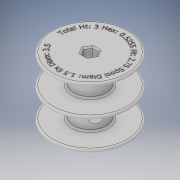
# Autodesk Inventor part: spoolV01
Saved by Autodesk Inventor 2019.3 (Build 233278000, 278)
## iProperties
Created: 2019-02-25
Part Number: spoolV01
Material: Generic
Document SubType Name: Modeling
Designer: steele
Density: 1 g/cm^3
Appearance: Default
d0: 2.750 in
d1: 0.150 in
d2: 0.750 in
d3: 1.750 in
d4: 0.075 in
d5: 0.075 in
d8: 0.523 in
d10: 0.00 deg
d17: 0.575 in
d18: 0.575 in
d19: 0.200 in
d20: 0.361 in
d21: 0.361 in
d23: 0.00 deg
d30: 2.625 in
d31: 0.050 in
d32: 0.00 deg
d33: 0.188 in
d36: 0.950 in
d37: 0.250 in
d38: 0.00 deg
d39: 0.063 in
holeForString: 0.200 in
stringDiameter: 0.120 in
clearanceForString: 0.080 in
hexShaftDiameter: 0.500 in
clearanceForHexShaft: 0.023 in
hexDiameter: 0.523 in
supportChannels: 0.150 in
spoolInteriorDiameter: 1.500 in
spoolInteriroRadius: 0.750 in
spoolExteriorDiameter: 3.500 in
spoolExteriorRadius: 1.750 in
spoolFiletRadius: 0.075 in
holeCenter: 0.575 in
hexHoleChamfer: 0.063 in
stringHoleCenterFromHexShaft: 0.361 in
textCircleDiameter: 2.625 in
textHeight: 0.240 in
textDepth: 0.050 in
stringHoleChamfer: 0.188 in
spoolTotalHeight: 3.000 in
spaceHeight: 0.250 in
spacerDiameter: 0.950 in
spoolHeightWithoutSpacer: 2.750 in
Author: steele
Autodesk Inventor part; units mm, degrees
(part 1 of 2)
ref_plane "YZ Plane" through (0, 0, 0) normal (1, 0, 0) x (0, 1, 0)
ref_plane "XZ Plane" through (0, 0, 0) normal (0, 1, 0) x (-1, 0, 0)
sketch "Sketch1" plane through (0, 0, 0) normal (1, 0, 0) x (0, 1, 0)
  line L0 (0, 0) -> (0, -42.545)
  line L1 (1.905, -44.45) -> (1.905, -44.45)
  line L2 (3.81, -42.545) -> (3.81, -20.955)
  line L3 (5.715, -19.05) -> (31.115, -19.05)
  line L4 (33.02, -20.955) -> (33.02, -42.545)
  line L5 (34.925, -44.45) -> (34.925, -44.45)
  line L6 (36.83, -42.545) -> (36.83, -20.955)
  line L7 (38.735, -19.05) -> (64.135, -19.05)
  line L8 (66.04, -20.955) -> (66.04, -42.545)
  line L9 (67.945, -44.45) -> (67.945, -44.45)
  line L10 (69.85, -42.545) -> (69.85, 0)
  line L11 (0, 0) -> (69.85, 0)
  arc A0 (67.945, -44.45) -> (69.85, -42.545) centre (67.945, -42.545) ccw
  arc A1 (66.04, -42.545) -> (67.945, -44.45) centre (67.945, -42.545) ccw
  arc A2 (34.925, -44.45) -> (36.83, -42.545) centre (34.925, -42.545) ccw
  arc A3 (33.02, -42.545) -> (34.925, -44.45) centre (34.925, -42.545) ccw
  arc A4 (1.905, -44.45) -> (3.81, -42.545) centre (1.905, -42.545) ccw
  arc A5 (0, -42.545) -> (1.905, -44.45) centre (1.905, -42.545) ccw
  arc A6 (66.04, -20.955) -> (64.135, -19.05) centre (64.135, -20.955) ccw
  arc A7 (38.735, -19.05) -> (36.83, -20.955) centre (38.735, -20.955) ccw
  arc A8 (33.02, -20.955) -> (31.115, -19.05) centre (31.115, -20.955) ccw
  arc A9 (5.715, -19.05) -> (3.81, -20.955) centre (5.715, -20.955) ccw
  point P0 (66.04, -44.45)
  point P1 (69.85, -44.45)
  dimension "d0" = 69.85
  dimension "d1" = 3.81
  dimension "d2" = 19.05
  dimension "d3" = 44.45
  dimension "d4" = 1.905
  dimension "d5" = 1.905
  constraints: 24 end point, 20 point on circle, 20 tangent, 10 centre point, 8 equal radius, 6 perpendicular, 6 point on line, 5 collinear, 1 horizontal, 1 parallel, 1 vertical
  measures "d0" distance between parallel lines of L10 L0
  measures "d1" distance of point (66.04, -44.45) point (69.85, -44.45)
  measures "d2" distance between parallel lines of L3 L11
  measures "d3" distance between parallel lines of L1 L11
  measures "d4" radius of A0
  measures "d5" radius of A6
revolve "Revolution1" add sketch "Sketch1" angle 360 about axis through (0, 0, 0) along (0, 1, 0)
sketch "Sketch6" plane through (0, 0, 0) normal (0, -1, 0) x (1, 0, 0)
  circle A0 centre (0, 0) radius 12.065
  dimension "d36" = 24.13
  constraints: 1 centre point, 1 coincident
  measures "d36" diameter of A0
extrude "Spacer" add sketch "Sketch6" along normal blind 6.35
sketch "Sketch2" plane through (0, 69.85, 0) normal (0, 1, 0) x (1, 0, 0)
  line L0 (7.6623, 0) -> (3.8312, -6.6357)
  line L1 (3.8312, -6.6357) -> (-3.8312, -6.6357)
  line L2 (-3.8312, -6.6357) -> (-7.6623, 0)
  line L3 (-7.6623, 0) -> (-3.8312, 6.6357)
  line L4 (-3.8312, 6.6357) -> (3.8312, 6.6358)
  line L5 (3.8312, 6.6358) -> (7.6623, 0)
  point P0 (0, 0)
  point P1 (0, 0)
  dimension "d8" = 13.2715
  constraints: 12 end point, 1 coincident, 1 horizontal, 13 other
  measures "d8" distance between parallel lines of L1 L4
extrude "HexHole" cut sketch "Sketch2" along normal through all both and the other way through all
sketch "Sketch4" plane through (0, 0, 0) normal (1, 0, 0) x (0, 1, 0)
  circle A0 centre (51.435, 9.1758) radius 2.54
  circle A1 centre (18.415, 9.1758) radius 2.54
  line L0 (3.81, 42.545) -> (3.81, -42.545) projected
  line L1 (66.04, 42.545) -> (66.04, -42.545) projected
  line L2 (69.85, 0) -> (0, 0) projected
  dimension "d17" = 14.605
  dimension "d18" = 14.605
  dimension "d19" = 5.08
  dimension "d20" = 9.1758
  dimension "d21" = 9.1758
  constraints: 2 centre point, 1 equal radius
  measures "d17" distance from line of A1.centre L0
  measures "d18" distance from line of A0.centre L1
  measures "d19" diameter of A0
  measures "d20" distance from line of A1.centre L2
  measures "d21" distance from line of A0.centre L2
extrude "StringHoles" cut sketch "Sketch4" along normal through all both and the other way through all
sketch "Sketch5" plane through (0, 69.85, 0) normal (0, 1, 0) x (1, 0, 0)
  circle A0 centre (0, 0) radius 33.3375
  line L0 (-33.296, 1.697) -> (-37.7666, 1.9708)
  line L1 (-37.7666, 1.9708) -> (-37.8708, 0.2697)
  line L2 (-37.8708, 0.2697) -> (-38.4707, 0.3065)
  line L3 (-38.4707, 0.3065) -> (-38.2211, 4.3826)
  line L4 (-38.2211, 4.3826) -> (-37.6212, 4.3458)
  line L5 (-37.6212, 4.3458) -> (-37.7253, 2.6447)
  line L6 (-37.7253, 2.6447) -> (-33.2548, 2.3709)
  line L7 (-33.2548, 2.3709) -> (-33.296, 1.697)
  spline S0 degree 2 poles (-34.3762, 7.9551) (-33.4283, 7.7835) (-32.5604, 6.685) (-32.6983, 5.9234) knots 0 0 0 1 2 2 2
  spline S1 degree 2 poles (-32.6983, 5.9234) (-32.8398, 5.1416) (-34.0673, 4.4393) (-34.9828, 4.6051) knots 0 0 0 1 2 2 2
  spline S2 degree 2 poles (-34.9828, 4.6051) (-35.9226, 4.7753) (-36.7964, 5.8874) (-36.66, 6.6408) knots 0 0 0 1 2 2 2
  spline S3 degree 2 poles (-36.66, 6.6408) (-36.5221, 7.4024) (-35.32, 8.126) (-34.3762, 7.9551) knots 0 0 0 1 2 2 2
  spline S4 degree 2 poles (-34.4943, 7.3029) (-35.2234, 7.435) (-36.0284, 7.0327) (-36.1172, 6.5425) knots 0 0 0 1 2 2 2
  spline S5 degree 2 poles (-36.1172, 6.5425) (-36.2059, 6.0524) (-35.5939, 5.3893) (-34.8647, 5.2573) knots 0 0 0 1 2 2 2
  spline S6 degree 2 poles (-34.8647, 5.2573) (-34.1558, 5.1289) (-33.3298, 5.5316) (-33.2411, 6.0217) knots 0 0 0 1 2 2 2
  spline S7 degree 2 poles (-33.2411, 6.0217) (-33.1531, 6.5078) (-33.7732, 7.1724) (-34.4943, 7.3029) knots 0 0 0 1 2 2 2
  spline S8 degree 2 poles (-31.9292, 9.337) (-32.0692, 8.8333) (-32.8019, 8.4259) (-33.4246, 8.5989) knots 0 0 0 1 2 2 2
  line L8 (-33.4246, 8.5989) -> (-35.4594, 9.1643)
  line L9 (-35.4594, 9.1643) -> (-35.5751, 8.7478)
  line L10 (-35.5751, 8.7478) -> (-36.0868, 8.89)
  line L11 (-36.0868, 8.89) -> (-35.9711, 9.3064)
  line L12 (-35.9711, 9.3064) -> (-37.0262, 9.5996)
  line L13 (-37.0262, 9.5996) -> (-36.8542, 10.2183)
  line L14 (-36.8542, 10.2183) -> (-35.7992, 9.9252)
  line L15 (-35.7992, 9.9252) -> (-35.4829, 11.0636)
  line L16 (-35.4829, 11.0636) -> (-34.9712, 10.9214)
  line L17 (-34.9712, 10.9214) -> (-35.2875, 9.783)
  line L18 (-35.2875, 9.783) -> (-33.5383, 9.297)
  spline S9 degree 2 poles (-33.5383, 9.297) (-33.2606, 9.2199) (-32.9497, 9.1549) (-32.8001, 9.1859) knots 0 0 0 1 2 2 2
  spline S10 degree 2 poles (-32.8001, 9.1859) (-32.6696, 9.2095) (-32.4852, 9.4274) (-32.4257, 9.6416) knots 0 0 0 1 2 2 2
  spline S11 degree 2 poles (-32.4257, 9.6416) (-32.3838, 9.7923) (-32.3968, 10.0993) (-32.4069, 10.1705) knots 0 0 0 1 2 2 2
  line L19 (-32.4069, 10.1705) -> (-32.397, 10.2062)
  line L20 (-32.397, 10.2062) -> (-31.8417, 10.0519)
  spline S12 degree 2 poles (-31.8417, 10.0519) (-31.8426, 9.8641) (-31.8862, 9.4917) (-31.9292, 9.337) knots 0 0 0 1 2 2 2
  spline S13 degree 2 poles (-31.2991, 12.625) (-31.2728, 12.5315) (-31.1733, 12.2123) (-31.1591, 12.0749) knots 0 0 0 1 2 2 2
  spline S14 degree 2 poles (-31.1591, 12.0749) (-31.134, 11.885) (-31.1574, 11.555) (-31.2592, 11.2854) knots 0 0 0 1 2 2 2
  spline S15 degree 2 poles (-31.2592, 11.2854) (-31.3421, 11.0659) (-31.6575, 10.7318) (-31.8644, 10.6383) knots 0 0 0 1 2 2 2
  spline S16 degree 2 poles (-31.8644, 10.6383) (-32.0645, 10.551) (-32.5613, 10.5406) (-32.8001, 10.6307) knots 0 0 0 1 2 2 2
  spline S17 degree 2 poles (-32.8001, 10.6307) (-33.1698, 10.7703) (-33.5758, 11.2801) (-33.598, 11.6757) knots 0 0 0 1 2 2 2
  spline S18 degree 2 poles (-33.598, 11.6757) (-33.6233, 12.0284) (-33.419, 12.8842) (-33.2671, 13.3681) knots 0 0 0 1 2 2 2
  line L21 (-33.2671, 13.3681) -> (-33.3826, 13.4117)
  spline S19 degree 2 poles (-33.3826, 13.4117) (-33.5906, 13.4902) (-33.8966, 13.4605) (-34.0134, 13.3726) knots 0 0 0 1 2 2 2
  spline S20 degree 2 poles (-34.0134, 13.3726) (-34.1302, 13.2847) (-34.3015, 12.971) (-34.3684, 12.7938) knots 0 0 0 1 2 2 2
  spline S21 degree 2 poles (-34.3684, 12.7938) (-34.4469, 12.5858) (-34.536, 11.977) (-34.5227, 11.6508) knots 0 0 0 1 2 2 2
  line L22 (-34.5227, 11.6508) -> (-34.5358, 11.6161)
  line L23 (-34.5358, 11.6161) -> (-35.1482, 11.8473)
  spline S22 degree 2 poles (-35.1482, 11.8473) (-35.1319, 12.0304) (-35.0133, 12.6941) (-34.8984, 12.9983) knots 0 0 0 1 2 2 2
  spline S23 degree 2 poles (-34.8984, 12.9983) (-34.7588, 13.3681) (-34.4528, 13.8289) (-34.227, 13.9725) knots 0 0 0 1 2 2 2
  spline S24 degree 2 poles (-34.227, 13.9725) (-34.0064, 14.1137) (-33.4677, 14.1303) (-33.1327, 14.0038) knots 0 0 0 1 2 2 2
  line L24 (-33.1327, 14.0038) -> (-30.6948, 13.0833)
  line L25 (-30.6948, 13.0833) -> (-30.9216, 12.4825)
  line L26 (-30.9216, 12.4825) -> (-31.2991, 12.625)
  line L27 (-31.7997, 12.814) -> (-32.7895, 13.1878)
  spline S25 degree 2 poles (-32.7895, 13.1878) (-32.8517, 12.9648) (-33.032, 12.2892) (-33.0474, 12.0618) knots 0 0 0 1 2 2 2
  spline S26 degree 2 poles (-33.0474, 12.0618) (-33.0644, 11.7954) (-32.8779, 11.3686) (-32.6083, 11.2668) knots 0 0 0 1 2 2 2
  spline S27 degree 2 poles (-32.6083, 11.2668) (-32.3002, 11.1505) (-31.8574, 11.3793) (-31.7323, 11.7105) knots 0 0 0 1 2 2 2
  spline S28 degree 2 poles (-31.7323, 11.7105) (-31.6262, 11.9917) (-31.6943, 12.5454) (-31.7997, 12.814) knots 0 0 0 1 2 2 2
  line L28 (-30.0264, 14.4882) -> (-30.2999, 13.9071)
  line L29 (-30.2999, 13.9071) -> (-35.1011, 16.167)
  line L30 (-35.1011, 16.167) -> (-34.8276, 16.748)
  line L31 (-34.8276, 16.748) -> (-30.0264, 14.4882)
  line L32 (-26.4744, 20.3444) -> (-26.8556, 19.7872)
  line L33 (-26.8556, 19.7872) -> (-28.9078, 21.1911)
  line L34 (-28.9078, 21.1911) -> (-30.228, 19.2611)
  line L35 (-30.228, 19.2611) -> (-28.1758, 17.8573)
  line L36 (-28.1758, 17.8573) -> (-28.5569, 17.3)
  line L37 (-28.5569, 17.3) -> (-32.7498, 20.1682)
  line L38 (-32.7498, 20.1682) -> (-32.3686, 20.7254)
  line L39 (-32.3686, 20.7254) -> (-30.7241, 19.6005)
  line L40 (-30.7241, 19.6005) -> (-29.4039, 21.5304)
  line L41 (-29.4039, 21.5304) -> (-31.0484, 22.6554)
  line L42 (-31.0484, 22.6554) -> (-30.6673, 23.2126)
  line L43 (-30.6673, 23.2126) -> (-26.4744, 20.3444)
  spline S29 degree 2 poles (-25.029, 21.9136) (-25.3681, 21.5156) (-26.2042, 21.4546) (-26.6962, 21.8738) knots 0 0 0 1 2 2 2
  line L44 (-26.6962, 21.8738) -> (-28.3037, 23.2433)
  line L45 (-28.3037, 23.2433) -> (-28.5841, 22.9143)
  line L46 (-28.5841, 22.9143) -> (-28.9883, 23.2587)
  line L47 (-28.9883, 23.2587) -> (-28.708, 23.5877)
  line L48 (-28.708, 23.5877) -> (-29.5415, 24.2979)
  line L49 (-29.5415, 24.2979) -> (-29.125, 24.7867)
  line L50 (-29.125, 24.7867) -> (-28.2915, 24.0766)
  line L51 (-28.2915, 24.0766) -> (-27.5253, 24.9759)
  line L52 (-27.5253, 24.9759) -> (-27.121, 24.6315)
  line L53 (-27.121, 24.6315) -> (-27.8872, 23.7322)
  line L54 (-27.8872, 23.7322) -> (-26.5053, 22.5548)
  spline S30 degree 2 poles (-26.5053, 22.5548) (-26.286, 22.3679) (-26.0313, 22.178) (-25.8825, 22.1432) knots 0 0 0 1 2 2 2
  spline S31 degree 2 poles (-25.8825, 22.1432) (-25.7543, 22.1097) (-25.4952, 22.2296) (-25.3511, 22.3989) knots 0 0 0 1 2 2 2
  spline S32 degree 2 poles (-25.3511, 22.3989) (-25.2496, 22.5179) (-25.1321, 22.8018) (-25.1113, 22.8707) knots 0 0 0 1 2 2 2
  line L55 (-25.1113, 22.8707) -> (-25.0873, 22.8989)
  line L56 (-25.0873, 22.8989) -> (-24.6486, 22.5251)
  spline S33 degree 2 poles (-24.6486, 22.5251) (-24.7285, 22.3552) (-24.9249, 22.0358) (-25.029, 21.9136) knots 0 0 0 1 2 2 2
  line L57 (-23.4674, 23.6819) -> (-24.0394, 23.1012)
  line L58 (-24.0394, 23.1012) -> (-24.7316, 23.7829)
  line L59 (-24.7316, 23.7829) -> (-24.1597, 24.3636)
  line L60 (-24.1597, 24.3636) -> (-23.4674, 23.6819)
  line L61 (-25.4913, 25.675) -> (-26.0633, 25.0943)
  line L62 (-26.0633, 25.0943) -> (-26.7555, 25.7759)
  line L63 (-26.7555, 25.7759) -> (-26.1836, 26.3567)
  line L64 (-26.1836, 26.3567) -> (-25.4913, 25.675)
  spline S34 degree 2 poles (-22.5898, 30.4771) (-22.7391, 30.3675) (-22.9808, 30.0776) (-23.0821, 29.9164) knots 0 0 0 1 2 2 2
  spline S35 degree 2 poles (-23.0821, 29.9164) (-23.1733, 29.7625) (-23.2814, 29.4993) (-23.3187, 29.3901) knots 0 0 0 1 2 2 2
  line L65 (-23.3187, 29.3901) -> (-23.3519, 29.3658)
  line L66 (-23.3519, 29.3658) -> (-23.7783, 29.9464)
  spline S36 degree 2 poles (-23.7783, 29.9464) (-23.6698, 30.1742) (-23.1706, 30.781) (-22.8952, 30.9833) knots 0 0 0 1 2 2 2
  spline S37 degree 2 poles (-22.8952, 30.9833) (-22.6165, 31.188) (-22.1189, 31.3798) (-21.862, 31.3846) knots 0 0 0 1 2 2 2
  spline S38 degree 2 poles (-21.862, 31.3846) (-21.5877, 31.3868) (-21.1266, 31.1484) (-20.9414, 30.8962) knots 0 0 0 1 2 2 2
  spline S39 degree 2 poles (-20.9414, 30.8962) (-20.6928, 30.5578) (-20.7621, 29.7203) (-21.0252, 29.4249) knots 0 0 0 1 2 2 2
  line L67 (-21.0252, 29.4249) -> (-20.996, 29.385)
  spline S40 degree 2 poles (-20.996, 29.385) (-20.8471, 29.4535) (-20.4641, 29.551) (-20.2503, 29.5241) knots 0 0 0 1 2 2 2
  spline S41 degree 2 poles (-20.2503, 29.5241) (-20.0389, 29.5006) (-19.6067, 29.246) (-19.4093, 28.9773) knots 0 0 0 1 2 2 2
  spline S42 degree 2 poles (-19.4093, 28.9773) (-19.207, 28.7019) (-19.0525, 28.0951) (-19.0935, 27.7893) knots 0 0 0 1 2 2 2
  spline S43 degree 2 poles (-19.0935, 27.7893) (-19.1361, 27.4719) (-19.5024, 26.9066) (-19.8243, 26.6702) knots 0 0 0 1 2 2 2
  spline S44 degree 2 poles (-19.8243, 26.6702) (-20.1328, 26.4435) (-20.8463, 26.1493) (-21.1276, 26.1011) knots 0 0 0 1 2 2 2
  line L68 (-21.1276, 26.1011) -> (-21.5541, 26.6817)
  line L69 (-21.5541, 26.6817) -> (-21.5143, 26.7109)
  spline S45 degree 2 poles (-21.5143, 26.7109) (-21.2491, 26.7116) (-20.4946, 26.9082) (-20.2059, 27.1203) knots 0 0 0 1 2 2 2
  spline S46 degree 2 poles (-20.2059, 27.1203) (-20.0367, 27.2445) (-19.7763, 27.5993) (-19.7536, 27.8049) knots 0 0 0 1 2 2 2
  spline S47 degree 2 poles (-19.7536, 27.8049) (-19.7343, 28.0081) (-19.8327, 28.3854) (-19.9959, 28.6077) knots 0 0 0 1 2 2 2
  spline S48 degree 2 poles (-19.9959, 28.6077) (-20.1592, 28.83) (-20.5006, 29.0236) (-20.6777, 29.0212) knots 0 0 0 1 2 2 2
  spline S49 degree 2 poles (-20.6777, 29.0212) (-20.8547, 29.0189) (-21.2162, 28.8504) (-21.402, 28.7139) knots 0 0 0 1 2 2 2
  line L70 (-21.402, 28.7139) -> (-21.6343, 28.5433)
  line L71 (-21.6343, 28.5433) -> (-21.9681, 28.9979)
  line L72 (-21.9681, 28.9979) -> (-21.7857, 29.1319)
  spline S50 degree 2 poles (-21.7857, 29.1319) (-21.4174, 29.4024) (-21.2112, 30.0953) (-21.4573, 30.4304) knots 0 0 0 1 2 2 2
  spline S51 degree 2 poles (-21.4573, 30.4304) (-21.5719, 30.5863) (-21.8546, 30.7209) (-21.9995, 30.7166) knots 0 0 0 1 2 2 2
  spline S52 degree 2 poles (-21.9995, 30.7166) (-22.1536, 30.7107) (-22.4472, 30.5819) (-22.5898, 30.4771) knots 0 0 0 1 2 2 2
  line L73 (-12.5415, 30.9435) -> (-13.1522, 30.6558)
  line L74 (-13.1522, 30.6558) -> (-14.2121, 32.905)
  line L75 (-14.2121, 32.905) -> (-16.3273, 31.9084)
  line L76 (-16.3273, 31.9084) -> (-15.2674, 29.6591)
  line L77 (-15.2674, 29.6591) -> (-15.8782, 29.3713)
  line L78 (-15.8782, 29.3713) -> (-18.0435, 33.9667)
  line L79 (-18.0435, 33.9667) -> (-17.4327, 34.2545)
  line L80 (-17.4327, 34.2545) -> (-16.5835, 32.4521)
  line L81 (-16.5835, 32.4521) -> (-14.4682, 33.4488)
  line L82 (-14.4682, 33.4488) -> (-15.3175, 35.2512)
  line L83 (-15.3175, 35.2512) -> (-14.7068, 35.5389)
  line L84 (-14.7068, 35.5389) -> (-12.5415, 30.9435)
  spline S53 degree 2 poles (-10.0214, 31.7062) (-10.8904, 31.4234) (-12.1628, 32.0873) (-12.4558, 32.9877) knots 0 0 0 1 2 2 2
  spline S54 degree 2 poles (-12.4558, 32.9877) (-12.7437, 33.8724) (-12.1573, 35.2234) (-11.4096, 35.4667) knots 0 0 0 1 2 2 2
  spline S55 degree 2 poles (-11.4096, 35.4667) (-11.073, 35.5763) (-10.4886, 35.55) (-10.2293, 35.4049) knots 0 0 0 1 2 2 2
  spline S56 degree 2 poles (-10.2293, 35.4049) (-9.9661, 35.2612) (-9.5637, 34.7297) (-9.4223, 34.2952) knots 0 0 0 1 2 2 2
  line L85 (-9.4223, 34.2952) -> (-9.314, 33.9625)
  line L86 (-9.314, 33.9625) -> (-11.8233, 33.1459)
  spline S57 degree 2 poles (-11.8233, 33.1459) (-11.6182, 32.5156) (-10.7662, 32.0526) (-10.2024, 32.2361) knots 0 0 0 1 2 2 2
  spline S58 degree 2 poles (-10.2024, 32.2361) (-10.0028, 32.301) (-9.6446, 32.5172) (-9.5109, 32.6386) knots 0 0 0 1 2 2 2
  spline S59 degree 2 poles (-9.5109, 32.6386) (-9.372, 32.7704) (-9.1895, 32.9813) (-9.1355, 33.0681) knots 0 0 0 1 2 2 2
  line L87 (-9.1355, 33.0681) -> (-9.1003, 33.0796)
  line L88 (-9.1003, 33.0796) -> (-8.8837, 32.4141)
  spline S60 degree 2 poles (-8.8837, 32.4141) (-8.9754, 32.3367) (-9.2556, 32.1069) (-9.3694, 32.0309) knots 0 0 0 1 2 2 2
  spline S61 degree 2 poles (-9.3694, 32.0309) (-9.529, 31.9227) (-9.8021, 31.7776) (-10.0214, 31.7062) knots 0 0 0 1 2 2 2
  spline S62 degree 2 poles (-10.0606, 34.2347) (-10.1487, 34.4788) (-10.3677, 34.8058) (-10.505, 34.8953) knots 0 0 0 1 2 2 2
  spline S63 degree 2 poles (-10.505, 34.8953) (-10.6553, 34.9979) (-11.0352, 35.0345) (-11.2818, 34.9542) knots 0 0 0 1 2 2 2
  spline S64 degree 2 poles (-11.2818, 34.9542) (-11.5245, 34.8752) (-11.818, 34.6195) (-11.913, 34.4328) knots 0 0 0 1 2 2 2
  spline S65 degree 2 poles (-11.913, 34.4328) (-12.0029, 34.2433) (-12.0304, 33.8491) (-11.9749, 33.6117) knots 0 0 0 1 2 2 2
  line L89 (-11.9749, 33.6117) -> (-10.0606, 34.2347)
  line L90 (-5.2154, 32.9707) -> (-5.9848, 32.8085)
  line L91 (-5.9848, 32.8085) -> (-7.1866, 34.0193)
  line L92 (-7.1866, 34.0193) -> (-7.8217, 32.4214)
  line L93 (-7.8217, 32.4214) -> (-8.5347, 32.2711)
  line L94 (-8.5347, 32.2711) -> (-7.6313, 34.3926)
  line L95 (-7.6313, 34.3926) -> (-9.3087, 36.0038)
  line L96 (-9.3087, 36.0038) -> (-8.5393, 36.1659)
  line L97 (-8.5393, 36.1659) -> (-7.3441, 34.9664)
  line L98 (-7.3441, 34.9664) -> (-6.7146, 36.5505)
  line L99 (-6.7146, 36.5505) -> (-6.0016, 36.7008)
  line L100 (-6.0016, 36.7008) -> (-6.8986, 34.5891)
  line L101 (-6.8986, 34.5891) -> (-5.2154, 32.9707)
  line L102 (-3.5488, 33.1506) -> (-4.3582, 33.0539)
  line L103 (-4.3582, 33.0539) -> (-4.4734, 34.0186)
  line L104 (-4.4734, 34.0186) -> (-3.664, 34.1153)
  line L105 (-3.664, 34.1153) -> (-3.5488, 33.1506)
  line L106 (-3.8857, 35.9711) -> (-4.695, 35.8744)
  line L107 (-4.695, 35.8744) -> (-4.8103, 36.8391)
  line L108 (-4.8103, 36.8391) -> (-4.0009, 36.9357)
  line L109 (-4.0009, 36.9357) -> (-3.8857, 35.9711)
  spline S66 degree 2 poles (3.0843, 35.7816) (3.0287, 34.416) (2.1828, 33.1691) (1.356, 33.2028) knots 0 0 0 1 2 2 2
  spline S67 degree 2 poles (1.356, 33.2028) (0.5169, 33.237) (-0.2156, 34.5729) (-0.1612, 35.9097) knots 0 0 0 1 2 2 2
  spline S68 degree 2 poles (-0.1612, 35.9097) (-0.1053, 37.2835) (0.7404, 38.5222) (1.5712, 38.4884) knots 0 0 0 1 2 2 2
  spline S69 degree 2 poles (1.5712, 38.4884) (2.4062, 38.4544) (3.1383, 37.1061) (3.0843, 35.7816) knots 0 0 0 1 2 2 2
  spline S70 degree 2 poles (2.1494, 34.2706) (2.2583, 34.5174) (2.372, 35.2874) (2.3933, 35.8098) knots 0 0 0 1 2 2 2
  spline S71 degree 2 poles (2.3933, 35.8098) (2.4146, 36.3322) (2.3636, 37.1047) (2.2714, 37.368) knots 0 0 0 1 2 2 2
  spline S72 degree 2 poles (2.2714, 37.368) (2.1791, 37.6313) (1.8321, 37.9133) (1.5483, 37.9248) knots 0 0 0 1 2 2 2
  spline S73 degree 2 poles (1.5483, 37.9248) (1.2645, 37.9364) (0.8875, 37.6839) (0.7697, 37.4209) knots 0 0 0 1 2 2 2
  spline S74 degree 2 poles (0.7697, 37.4209) (0.6563, 37.166) (0.5501, 36.3792) (0.5298, 35.8815) knots 0 0 0 1 2 2 2
  spline S75 degree 2 poles (0.5298, 35.8815) (0.5081, 35.3468) (0.5447, 34.6284) (0.6403, 34.3444) knots 0 0 0 1 2 2 2
  spline S76 degree 2 poles (0.6403, 34.3444) (0.7283, 34.0771) (1.0828, 33.7784) (1.379, 33.7663) knots 0 0 0 1 2 2 2
  spline S77 degree 2 poles (1.379, 33.7663) (1.6587, 33.7549) (2.0356, 34.0074) (2.1494, 34.2706) knots 0 0 0 1 2 2 2
  line L110 (4.7062, 33.0061) -> (3.8979, 33.1114)
  line L111 (3.8979, 33.1114) -> (4.0234, 34.0748)
  line L112 (4.0234, 34.0748) -> (4.8317, 33.9695)
  line L113 (4.8317, 33.9695) -> (4.7062, 33.0061)
  spline S78 degree 2 poles (9.0788, 33.7868) (8.9994, 33.4291) (8.6348, 32.8691) (8.3759, 32.6904) knots 0 0 0 1 2 2 2
  spline S79 degree 2 poles (8.3759, 32.6904) (8.1169, 32.5117) (7.436, 32.3887) (7.0502, 32.4743) knots 0 0 0 1 2 2 2
  spline S80 degree 2 poles (7.0502, 32.4743) (6.6966, 32.5528) (6.0401, 32.8629) (5.8145, 33.0437) knots 0 0 0 1 2 2 2
  line L114 (5.8145, 33.0437) -> (5.9706, 33.747)
  line L115 (5.9706, 33.747) -> (6.0188, 33.7363)
  spline S81 degree 2 poles (6.0188, 33.7363) (6.0827, 33.6631) (6.3359, 33.4551) (6.4945, 33.3525) knots 0 0 0 1 2 2 2
  spline S82 degree 2 poles (6.4945, 33.3525) (6.6763, 33.2404) (6.9848, 33.0918) (7.1898, 33.0464) knots 0 0 0 1 2 2 2
  spline S83 degree 2 poles (7.1898, 33.0464) (7.3908, 33.0018) (7.8006, 33.0626) (7.9721, 33.189) knots 0 0 0 1 2 2 2
  spline S84 degree 2 poles (7.9721, 33.189) (8.1296, 33.3101) (8.3457, 33.6754) (8.4045, 33.9406) knots 0 0 0 1 2 2 2
  spline S85 degree 2 poles (8.4045, 33.9406) (8.4634, 34.2059) (8.3936, 34.5756) (8.2819, 34.7184) knots 0 0 0 1 2 2 2
  spline S86 degree 2 poles (8.2819, 34.7184) (8.1689, 34.8742) (7.7741, 35.0715) (7.5209, 35.1277) knots 0 0 0 1 2 2 2
  spline S87 degree 2 poles (7.5209, 35.1277) (7.2477, 35.1883) (6.6864, 35.2243) (6.5136, 35.2247) knots 0 0 0 1 2 2 2
  line L116 (6.5136, 35.2247) -> (7.0808, 37.7808)
  line L117 (7.0808, 37.7808) -> (9.8016, 37.177)
  line L118 (9.8016, 37.177) -> (9.6723, 36.5942)
  line L119 (9.6723, 36.5942) -> (7.5905, 37.0562)
  line L120 (7.5905, 37.0562) -> (7.2971, 35.734)
  spline S88 degree 2 poles (7.2971, 35.734) (7.4212, 35.7233) (7.657, 35.6836) (7.7534, 35.6622) knots 0 0 0 1 2 2 2
  spline S89 degree 2 poles (7.7534, 35.6622) (8.1352, 35.5775) (8.634, 35.3361) (8.8342, 35.0977) knots 0 0 0 1 2 2 2
  spline S90 degree 2 poles (8.8342, 35.0977) (9.0383, 34.8584) (9.1787, 34.2369) (9.0788, 33.7868) knots 0 0 0 1 2 2 2
  line L121 (12.3942, 30.9891) -> (9.4331, 32.0119)
  line L122 (9.4331, 32.0119) -> (9.6683, 32.6929)
  spline S91 degree 2 poles (9.6683, 32.6929) (10.0908, 32.8823) (10.8511, 33.2425) (11.227, 33.448) knots 0 0 0 1 2 2 2
  spline S92 degree 2 poles (11.227, 33.448) (11.984, 33.8616) (12.6348, 34.4469) (12.7678, 34.8321) knots 0 0 0 1 2 2 2
  spline S93 degree 2 poles (12.7678, 34.8321) (12.8377, 35.0345) (12.8181, 35.381) (12.7388, 35.5172) knots 0 0 0 1 2 2 2
  spline S94 degree 2 poles (12.7388, 35.5172) (12.6596, 35.6535) (12.3974, 35.8529) (12.2185, 35.9147) knots 0 0 0 1 2 2 2
  spline S95 degree 2 poles (12.2185, 35.9147) (12.0473, 35.9739) (11.6675, 36.0092) (11.4851, 35.9982) knots 0 0 0 1 2 2 2
  spline S96 degree 2 poles (11.4851, 35.9982) (11.3301, 35.9908) (11.0234, 35.9225) (10.9268, 35.8949) knots 0 0 0 1 2 2 2
  line L123 (10.9268, 35.8949) -> (10.8917, 35.907)
  line L124 (10.8917, 35.907) -> (11.1283, 36.5918)
  spline S97 degree 2 poles (11.1283, 36.5918) (11.3604, 36.6206) (12.1383, 36.5653) (12.4574, 36.455) knots 0 0 0 1 2 2 2
  spline S98 degree 2 poles (12.4574, 36.455) (13.1305, 36.2225) (13.6433, 35.2484) (13.4336, 34.6413) knots 0 0 0 1 2 2 2
  spline S99 degree 2 poles (13.4336, 34.6413) (13.3355, 34.3573) (13.0392, 33.9283) (12.8526, 33.7663) knots 0 0 0 1 2 2 2
  spline S100 degree 2 poles (12.8526, 33.7663) (12.6633, 33.5965) (12.1823, 33.3009) (11.927, 33.167) knots 0 0 0 1 2 2 2
  spline S101 degree 2 poles (11.927, 33.167) (11.5092, 32.9411) (10.5214, 32.4896) (10.2284, 32.36) knots 0 0 0 1 2 2 2
  line L125 (10.2284, 32.36) -> (12.5864, 31.5455)
  line L126 (12.5864, 31.5455) -> (12.3942, 30.9891)
  spline S102 degree 2 poles (16.4944, 30.853) (16.3361, 30.5226) (15.8541, 30.0596) (15.5615, 29.9442) knots 0 0 0 1 2 2 2
  spline S103 degree 2 poles (15.5615, 29.9442) (15.2688, 29.8288) (14.5777, 29.8632) (14.2213, 30.034) knots 0 0 0 1 2 2 2
  spline S104 degree 2 poles (14.2213, 30.034) (13.8946, 30.1905) (13.3254, 30.6413) (13.1467, 30.8684) knots 0 0 0 1 2 2 2
  line L127 (13.1467, 30.8684) -> (13.458, 31.5181)
  line L128 (13.458, 31.5181) -> (13.5025, 31.4968)
  spline S105 degree 2 poles (13.5025, 31.4968) (13.5482, 31.411) (13.7477, 31.1511) (13.8789, 31.0152) knots 0 0 0 1 2 2 2
  spline S106 degree 2 poles (13.8789, 31.0152) (14.0306, 30.8649) (14.2975, 30.6503) (14.4868, 30.5596) knots 0 0 0 1 2 2 2
  spline S107 degree 2 poles (14.4868, 30.5596) (14.6725, 30.4706) (15.0855, 30.4371) (15.2811, 30.5214) knots 0 0 0 1 2 2 2
  spline S108 degree 2 poles (15.2811, 30.5214) (15.462, 30.6036) (15.7551, 30.9105) (15.8725, 31.1555) knots 0 0 0 1 2 2 2
  spline S109 degree 2 poles (15.8725, 31.1555) (15.9899, 31.4006) (16.0057, 31.7764) (15.9293, 31.9409) knots 0 0 0 1 2 2 2
  spline S110 degree 2 poles (15.9293, 31.9409) (15.8545, 32.1182) (15.5146, 32.3997) (15.2807, 32.5118) knots 0 0 0 1 2 2 2
  spline S111 degree 2 poles (15.2807, 32.5118) (15.0283, 32.6328) (14.4897, 32.7949) (14.3215, 32.8345) knots 0 0 0 1 2 2 2
  line L129 (14.3215, 32.8345) -> (15.4528, 35.1956)
  line L130 (15.4528, 35.1956) -> (17.9662, 33.9914)
  line L131 (17.9662, 33.9914) -> (17.7083, 33.4531)
  line L132 (17.7083, 33.4531) -> (15.7852, 34.3745)
  line L133 (15.7852, 34.3745) -> (15.1999, 33.1531)
  spline S112 degree 2 poles (15.1999, 33.1531) (15.3184, 33.1146) (15.5391, 33.0225) (15.6282, 32.9798) knots 0 0 0 1 2 2 2
  spline S113 degree 2 poles (15.6282, 32.9798) (15.9809, 32.8108) (16.4121, 32.4627) (16.553, 32.1852) knots 0 0 0 1 2 2 2
  spline S114 degree 2 poles (16.553, 32.1852) (16.6977, 31.9059) (16.6937, 31.2688) (16.4944, 30.853) knots 0 0 0 1 2 2 2
  spline S115 degree 2 poles (19.9034, 28.772) (19.7085, 28.4618) (19.1769, 28.0568) (18.873, 27.9755) knots 0 0 0 1 2 2 2
  spline S116 degree 2 poles (18.873, 27.9755) (18.569, 27.8942) (17.8864, 28.0071) (17.5518, 28.2174) knots 0 0 0 1 2 2 2
  spline S117 degree 2 poles (17.5518, 28.2174) (17.245, 28.4102) (16.7309, 28.9228) (16.5792, 29.1689) knots 0 0 0 1 2 2 2
  line L134 (16.5792, 29.1689) -> (16.9626, 29.7789)
  line L135 (16.9626, 29.7789) -> (17.0044, 29.7526)
  spline S118 degree 2 poles (17.0044, 29.7526) (17.0399, 29.6622) (17.2086, 29.3812) (17.3234, 29.2312) knots 0 0 0 1 2 2 2
  spline S119 degree 2 poles (17.3234, 29.2312) (17.457, 29.0646) (17.6977, 28.821) (17.8755, 28.7093) knots 0 0 0 1 2 2 2
  spline S120 degree 2 poles (17.8755, 28.7093) (18.0497, 28.5998) (18.4562, 28.5194) (18.6602, 28.5808) knots 0 0 0 1 2 2 2
  spline S121 degree 2 poles (18.6602, 28.5808) (18.8493, 28.6419) (19.1755, 28.9134) (19.32, 29.1434) knots 0 0 0 1 2 2 2
  spline S122 degree 2 poles (19.32, 29.1434) (19.4646, 29.3735) (19.5231, 29.7451) (19.4659, 29.9172) knots 0 0 0 1 2 2 2
  spline S123 degree 2 poles (19.4659, 29.9172) (19.4118, 30.1019) (19.1063, 30.4203) (18.8867, 30.5583) knots 0 0 0 1 2 2 2
  spline S124 degree 2 poles (18.8867, 30.5583) (18.6496, 30.7073) (18.1331, 30.9298) (17.9705, 30.9882) knots 0 0 0 1 2 2 2
  line L136 (17.9705, 30.9882) -> (19.3635, 33.2051)
  line L137 (19.3635, 33.2051) -> (21.7233, 31.7222)
  line L138 (21.7233, 31.7222) -> (21.4057, 31.2168)
  line L139 (21.4057, 31.2168) -> (19.6001, 32.3514)
  line L140 (19.6001, 32.3514) -> (18.8795, 31.2046)
  spline S125 degree 2 poles (18.8795, 31.2046) (18.9928, 31.1528) (19.2016, 31.0363) (19.2852, 30.9837) knots 0 0 0 1 2 2 2
  spline S126 degree 2 poles (19.2852, 30.9837) (19.6164, 30.7756) (20.0051, 30.3806) (20.1135, 30.0889) knots 0 0 0 1 2 2 2
  spline S127 degree 2 poles (20.1135, 30.0889) (20.2253, 29.7949) (20.1487, 29.1624) (19.9034, 28.772) knots 0 0 0 1 2 2 2
  line L141 (24.1708, 23.034) -> (23.6787, 23.4962)
  line L142 (23.6787, 23.4962) -> (25.3813, 25.3084)
  line L143 (25.3813, 25.3084) -> (23.6771, 26.9095)
  line L144 (23.6771, 26.9095) -> (21.9746, 25.0973)
  line L145 (21.9746, 25.0973) -> (21.4825, 25.5596)
  line L146 (21.4825, 25.5596) -> (24.9609, 29.2619)
  line L147 (24.9609, 29.2619) -> (25.4529, 28.7996)
  line L148 (25.4529, 28.7996) -> (24.0886, 27.3475)
  line L149 (24.0886, 27.3475) -> (25.7928, 25.7465)
  line L150 (25.7928, 25.7465) -> (27.1571, 27.1986)
  line L151 (27.1571, 27.1986) -> (27.6491, 26.7363)
  line L152 (27.6491, 26.7363) -> (24.1708, 23.034)
  spline S128 degree 2 poles (25.4992, 21.3646) (25.158, 21.7608) (25.2263, 22.5964) (25.716, 23.0181) knots 0 0 0 1 2 2 2
  line L153 (25.716, 23.0181) -> (27.3164, 24.3961)
  line L154 (27.3164, 24.3961) -> (27.0343, 24.7237)
  line L155 (27.0343, 24.7237) -> (27.4367, 25.0702)
  line L156 (27.4367, 25.0702) -> (27.7188, 24.7426)
  line L157 (27.7188, 24.7426) -> (28.5486, 25.4572)
  line L158 (28.5486, 25.4572) -> (28.9676, 24.9705)
  line L159 (28.9676, 24.9705) -> (28.1378, 24.256)
  line L160 (28.1378, 24.256) -> (28.9088, 23.3607)
  line L161 (28.9088, 23.3607) -> (28.5063, 23.0142)
  line L162 (28.5063, 23.0142) -> (27.7354, 23.9095)
  line L163 (27.7354, 23.9095) -> (26.3597, 22.7249)
  spline S129 degree 2 poles (26.3597, 22.7249) (26.1413, 22.5368) (25.9145, 22.3144) (25.8572, 22.1727) knots 0 0 0 1 2 2 2
  spline S130 degree 2 poles (25.8572, 22.1727) (25.8044, 22.0512) (25.8831, 21.7767) (26.0282, 21.6083) knots 0 0 0 1 2 2 2
  spline S131 degree 2 poles (26.0282, 21.6083) (26.1303, 21.4897) (26.3927, 21.33) (26.4576, 21.2989) knots 0 0 0 1 2 2 2
  line L164 (26.4576, 21.2989) -> (26.4817, 21.2708)
  line L165 (26.4817, 21.2708) -> (26.045, 20.8948)
  spline S132 degree 2 poles (26.045, 20.8948) (25.8894, 20.9998) (25.6039, 21.243) (25.4992, 21.3646) knots 0 0 0 1 2 2 2
  line L166 (27.0066, 19.5499) -> (26.5206, 20.2042)
  line L167 (26.5206, 20.2042) -> (27.3006, 20.7835)
  line L168 (27.3006, 20.7835) -> (27.7866, 20.1291)
  line L169 (27.7866, 20.1291) -> (27.0066, 19.5499)
  line L170 (29.287, 21.2435) -> (28.801, 21.8979)
  line L171 (28.801, 21.8979) -> (29.581, 22.4771)
  line L172 (29.581, 22.4771) -> (30.067, 21.8228)
  line L173 (30.067, 21.8228) -> (29.287, 21.2435)
  line L174 (30.3184, 13.9548) -> (28.8738, 16.7347)
  line L175 (28.8738, 16.7347) -> (29.5131, 17.0669)
  spline S133 degree 2 poles (29.5131, 17.0669) (29.95, 16.9135) (30.7495, 16.6516) (31.1637, 16.5421) knots 0 0 0 1 2 2 2
  spline S134 degree 2 poles (31.1637, 16.5421) (31.9975, 16.3212) (32.8725, 16.2981) (33.2341, 16.486) knots 0 0 0 1 2 2 2
  spline S135 degree 2 poles (33.2341, 16.486) (33.4241, 16.5847) (33.6483, 16.8496) (33.6845, 17.003) knots 0 0 0 1 2 2 2
  spline S136 degree 2 poles (33.6845, 17.003) (33.7208, 17.1564) (33.6679, 17.4815) (33.5806, 17.6495) knots 0 0 0 1 2 2 2
  spline S137 degree 2 poles (33.5806, 17.6495) (33.497, 17.8103) (33.2458, 18.0973) (33.1059, 18.2148) knots 0 0 0 1 2 2 2
  spline S138 degree 2 poles (33.1059, 18.2148) (32.9883, 18.316) (32.7188, 18.4776) (32.6297, 18.524) knots 0 0 0 1 2 2 2
  line L176 (32.6297, 18.524) -> (32.6126, 18.5569)
  line L177 (32.6126, 18.5569) -> (33.2555, 18.891)
  spline S139 degree 2 poles (33.2555, 18.891) (33.4437, 18.7522) (33.97, 18.1767) (34.1257, 17.8771) knots 0 0 0 1 2 2 2
  spline S140 degree 2 poles (34.1257, 17.8771) (34.4541, 17.2452) (34.1558, 16.1855) (33.5859, 15.8894) knots 0 0 0 1 2 2 2
  spline S141 degree 2 poles (33.5859, 15.8894) (33.3192, 15.7508) (32.809, 15.6434) (32.5622, 15.6543) knots 0 0 0 1 2 2 2
  spline S142 degree 2 poles (32.5622, 15.6543) (32.3079, 15.6614) (31.7556, 15.778) (31.4782, 15.8565) knots 0 0 0 1 2 2 2
  spline S143 degree 2 poles (31.4782, 15.8565) (31.0196, 15.9801) (29.9922, 16.3323) (29.6904, 16.4399) knots 0 0 0 1 2 2 2
  line L178 (29.6904, 16.4399) -> (30.8407, 14.2262)
  line L179 (30.8407, 14.2262) -> (30.3184, 13.9548)
  line L180 (30.9826, 12.3139) -> (30.6724, 13.0677)
  line L181 (30.6724, 13.0677) -> (31.5708, 13.4374)
  line L182 (31.5708, 13.4374) -> (31.881, 12.6837)
  line L183 (31.881, 12.6837) -> (30.9826, 12.3139)
  line L184 (36.4481, 9.6043) -> (31.6716, 10.4207)
  line L185 (31.6716, 10.4207) -> (31.4564, 11.1126)
  line L186 (31.4564, 11.1126) -> (36.4268, 10.2271)
  line L187 (36.4268, 10.2271) -> (35.6479, 12.7311)
  line L188 (35.6479, 12.7311) -> (36.2179, 12.9084)
  line L189 (36.2179, 12.9084) -> (37.1753, 9.8305)
  line L190 (37.1753, 9.8305) -> (36.4481, 9.6043)
  spline S144 degree 2 poles (34.6272, 4.993) (34.2672, 4.9247) (33.6087, 5.0387) (33.3424, 5.2061) knots 0 0 0 1 2 2 2
  spline S145 degree 2 poles (33.3424, 5.2061) (33.076, 5.3735) (32.6942, 5.9506) (32.6206, 6.3389) knots 0 0 0 1 2 2 2
  spline S146 degree 2 poles (32.6206, 6.3389) (32.5532, 6.6948) (32.579, 7.4204) (32.6561, 7.699) knots 0 0 0 1 2 2 2
  line L191 (32.6561, 7.699) -> (33.3639, 7.8331)
  line L192 (33.3639, 7.8331) -> (33.3731, 7.7846)
  spline S147 degree 2 poles (33.3731, 7.7846) (33.3311, 7.697) (33.2399, 7.3823) (33.2081, 7.1961) knots 0 0 0 1 2 2 2
  spline S148 degree 2 poles (33.2081, 7.1961) (33.177, 6.9848) (33.1622, 6.6427) (33.2013, 6.4364) knots 0 0 0 1 2 2 2
  spline S149 degree 2 poles (33.2013, 6.4364) (33.2397, 6.2341) (33.4573, 5.8815) (33.6412, 5.7739) knots 0 0 0 1 2 2 2
  spline S150 degree 2 poles (33.6412, 5.7739) (33.8146, 5.6769) (34.2355, 5.6226) (34.5024, 5.6732) knots 0 0 0 1 2 2 2
  spline S151 degree 2 poles (34.5024, 5.6732) (34.7694, 5.7238) (35.0815, 5.9339) (35.1687, 6.0928) knots 0 0 0 1 2 2 2
  spline S152 degree 2 poles (35.1687, 6.0928) (35.2673, 6.2582) (35.2927, 6.6988) (35.2444, 6.9536) knots 0 0 0 1 2 2 2
  spline S153 degree 2 poles (35.2444, 6.9536) (35.1922, 7.2286) (35.0038, 7.7585) (34.936, 7.9175) knots 0 0 0 1 2 2 2
  line L193 (34.936, 7.9175) -> (37.5084, 8.4051)
  line L194 (37.5084, 8.4051) -> (38.0274, 5.6669)
  line L195 (38.0274, 5.6669) -> (37.441, 5.5557)
  line L196 (37.441, 5.5557) -> (37.0438, 7.6508)
  line L197 (37.0438, 7.6508) -> (35.7131, 7.3986)
  spline S154 degree 2 poles (35.7131, 7.3986) (35.7523, 7.2803) (35.8089, 7.048) (35.8273, 6.9509) knots 0 0 0 1 2 2 2
  spline S155 degree 2 poles (35.8273, 6.9509) (35.9001, 6.5667) (35.8752, 6.0131) (35.7351, 5.7351) knots 0 0 0 1 2 2 2
  spline S156 degree 2 poles (35.7351, 5.7351) (35.5958, 5.4531) (35.0802, 5.0788) (34.6272, 4.993) knots 0 0 0 1 2 2 2
  spline S157 degree 2 poles (33.2461, 0.2315) (33.2425, 0.7831) (33.468, 1.5585) (33.6304, 1.9013) knots 0 0 0 1 2 2 2
  line L198 (33.6304, 1.9013) -> (34.4785, 1.9068)
  line L199 (34.4785, 1.9068) -> (34.4788, 1.8574)
  spline S158 degree 2 poles (34.4788, 1.8574) (34.1681, 1.5219) (33.8278, 0.6758) (33.8304, 0.2847) knots 0 0 0 1 2 2 2
  spline S159 degree 2 poles (33.8304, 0.2847) (33.834, -0.2752) (34.3029, -0.8443) (34.6858, -0.8418) knots 0 0 0 1 2 2 2
  spline S160 degree 2 poles (34.6858, -0.8418) (34.9904, -0.8398) (35.3672, -0.5369) (35.4597, -0.211) knots 0 0 0 1 2 2 2
  spline S161 degree 2 poles (35.4597, -0.211) (35.5241, 0.024) (35.6121, 0.4157) (35.6843, 0.7085) knots 0 0 0 1 2 2 2
  spline S162 degree 2 poles (35.6843, 0.7085) (35.7525, 0.9724) (35.9598, 1.3895) (36.1275, 1.5512) knots 0 0 0 1 2 2 2
  spline S163 degree 2 poles (36.1275, 1.5512) (36.2953, 1.7087) (36.747, 1.8846) (37.0433, 1.8865) knots 0 0 0 1 2 2 2
  spline S164 degree 2 poles (37.0433, 1.8865) (37.6608, 1.8905) (38.5028, 0.9327) (38.5077, 0.1876) knots 0 0 0 1 2 2 2
  spline S165 degree 2 poles (38.5077, 0.1876) (38.5105, -0.2405) (38.3466, -0.9991) (38.1882, -1.3253) knots 0 0 0 1 2 2 2
  line L200 (38.1882, -1.3253) -> (37.3813, -1.3306)
  line L201 (37.3813, -1.3306) -> (37.381, -1.2812)
  spline S166 degree 2 poles (37.381, -1.2812) (37.6017, -1.0369) (37.9261, -0.2773) (37.9234, 0.1385) knots 0 0 0 1 2 2 2
  spline S167 degree 2 poles (37.9234, 0.1385) (37.9203, 0.6078) (37.4761, 1.1854) (37.1179, 1.183) knots 0 0 0 1 2 2 2
  spline S168 degree 2 poles (37.1179, 1.183) (36.7968, 1.1809) (36.4162, 0.8368) (36.3319, 0.5151) knots 0 0 0 1 2 2 2
  spline S169 degree 2 poles (36.3319, 0.5151) (36.2756, 0.3007) (36.1315, -0.3219) (36.0711, -0.5282) knots 0 0 0 1 2 2 2
  spline S170 degree 2 poles (36.0711, -0.5282) (35.914, -1.052) (35.2708, -1.542) (34.7974, -1.5451) knots 0 0 0 1 2 2 2
  spline S171 degree 2 poles (34.7974, -1.5451) (34.4969, -1.547) (33.919, -1.3079) (33.7158, -1.0911) knots 0 0 0 1 2 2 2
  spline S172 degree 2 poles (33.7158, -1.0911) (33.492, -0.8496) (33.2492, -0.2337) (33.2461, 0.2315) knots 0 0 0 1 2 2 2
  spline S173 degree 2 poles (34.9452, -5.5849) (33.9959, -5.4805) (32.9742, -4.4527) (33.0503, -3.7612) knots 0 0 0 1 2 2 2
  spline S174 degree 2 poles (33.0503, -3.7612) (33.0814, -3.4788) (33.26, -3.0595) (33.4198, -2.8493) knots 0 0 0 1 2 2 2
  line L202 (33.4198, -2.8493) -> (31.8322, -2.6746)
  line L203 (31.8322, -2.6746) -> (31.9024, -2.0362)
  line L204 (31.9024, -2.0362) -> (37.087, -2.6068)
  line L205 (37.087, -2.6068) -> (37.0167, -3.2451)
  line L206 (37.0167, -3.2451) -> (36.6198, -3.2014)
  spline S175 degree 2 poles (36.6198, -3.2014) (36.8105, -3.4626) (37.033, -4.0752) (36.9957, -4.4149) knots 0 0 0 1 2 2 2
  spline S176 degree 2 poles (36.9957, -4.4149) (36.9241, -5.0655) (35.8127, -5.6804) (34.9452, -5.5849) knots 0 0 0 1 2 2 2
  spline S177 degree 2 poles (34.9441, -4.918) (35.5947, -4.9896) (36.3563, -4.6551) (36.4072, -4.1927) knots 0 0 0 1 2 2 2
  spline S178 degree 2 poles (36.4072, -4.1927) (36.4369, -3.9226) (36.2513, -3.3887) (36.0878, -3.1429) knots 0 0 0 1 2 2 2
  line L207 (36.0878, -3.1429) -> (33.9354, -2.906)
  spline S179 degree 2 poles (33.9354, -2.906) (33.7893, -3.1426) (33.6601, -3.4887) (33.6349, -3.7178) knots 0 0 0 1 2 2 2
  spline S180 degree 2 poles (33.6349, -3.7178) (33.5804, -4.213) (34.2484, -4.8415) (34.9441, -4.918) knots 0 0 0 1 2 2 2
  spline S181 degree 2 poles (33.9825, -9.4971) (33.0433, -9.2829) (32.2258, -8.1464) (32.3979, -7.3918) knots 0 0 0 1 2 2 2
  spline S182 degree 2 poles (32.3979, -7.3918) (32.5746, -6.6172) (33.8325, -5.971) (34.7396, -6.1779) knots 0 0 0 1 2 2 2
  spline S183 degree 2 poles (34.7396, -6.1779) (35.6707, -6.3902) (36.4935, -7.5406) (36.3232, -8.2872) knots 0 0 0 1 2 2 2
  spline S184 degree 2 poles (36.3232, -8.2872) (36.1511, -9.0417) (34.9177, -9.7104) (33.9825, -9.4971) knots 0 0 0 1 2 2 2
  spline S185 degree 2 poles (34.1299, -8.8509) (34.8523, -9.0157) (35.6746, -8.6501) (35.7854, -8.1645) knots 0 0 0 1 2 2 2
  spline S186 degree 2 poles (35.7854, -8.1645) (35.8962, -7.6788) (35.3146, -6.9888) (34.5922, -6.824) knots 0 0 0 1 2 2 2
  spline S187 degree 2 poles (34.5922, -6.824) (33.8898, -6.6638) (33.0465, -7.0288) (32.9357, -7.5145) knots 0 0 0 1 2 2 2
  spline S188 degree 2 poles (32.9357, -7.5145) (32.8259, -7.9961) (33.4154, -8.688) (34.1299, -8.8509) knots 0 0 0 1 2 2 2
  spline S189 degree 2 poles (32.6868, -13.2883) (31.7779, -12.9689) (31.0946, -11.7471) (31.3511, -11.0169) knots 0 0 0 1 2 2 2
  spline S190 degree 2 poles (31.3511, -11.0169) (31.6145, -10.2673) (32.9375, -9.7678) (33.8153, -10.0762) knots 0 0 0 1 2 2 2
  spline S191 degree 2 poles (33.8153, -10.0762) (34.7164, -10.3928) (35.4034, -11.629) (35.1496, -12.3515) knots 0 0 0 1 2 2 2
  spline S192 degree 2 poles (35.1496, -12.3515) (34.8931, -13.0816) (33.5918, -13.6062) (32.6868, -13.2883) knots 0 0 0 1 2 2 2
  spline S193 degree 2 poles (32.9065, -12.6629) (33.6056, -12.9086) (34.464, -12.6386) (34.6292, -12.1686) knots 0 0 0 1 2 2 2
  spline S194 degree 2 poles (34.6292, -12.1686) (34.7943, -11.6986) (34.2947, -10.9472) (33.5956, -10.7015) knots 0 0 0 1 2 2 2
  spline S195 degree 2 poles (33.5956, -10.7015) (32.9159, -10.4627) (32.0367, -10.7298) (31.8716, -11.1998) knots 0 0 0 1 2 2 2
  spline S196 degree 2 poles (31.8716, -11.1998) (31.7078, -11.6658) (32.2151, -12.42) (32.9065, -12.6629) knots 0 0 0 1 2 2 2
  line L208 (30.3283, -13.845) -> (30.5894, -13.2583)
  line L209 (30.5894, -13.2583) -> (35.4376, -15.4153)
  line L210 (35.4376, -15.4153) -> (35.1765, -16.0021)
  line L211 (35.1765, -16.0021) -> (30.3283, -13.845)
  spline S197 degree 2 poles (28.8507, -21.4281) (28.2683, -21.0475) (27.6396, -19.9627) (27.6368, -19.3953) knots 0 0 0 1 2 2 2
  spline S198 degree 2 poles (27.6368, -19.3953) (27.6452, -18.9385) (27.9421, -18.1833) (28.2799, -17.6665) knots 0 0 0 1 2 2 2
  line L212 (28.2799, -17.6665) -> (28.9196, -16.6878)
  line L213 (28.9196, -16.6878) -> (33.1718, -19.4673)
  line L214 (33.1718, -19.4673) -> (32.5389, -20.4356)
  spline S199 degree 2 poles (32.5389, -20.4356) (32.1469, -21.0352) (31.5218, -21.6003) (31.2056, -21.7379) knots 0 0 0 1 2 2 2
  spline S200 degree 2 poles (31.2056, -21.7379) (30.6654, -21.97) (29.4709, -21.8336) (28.8507, -21.4281) knots 0 0 0 1 2 2 2
  spline S201 degree 2 poles (29.2427, -20.8434) (29.732, -21.1632) (30.6364, -21.2921) (31.0423, -21.1) knots 0 0 0 1 2 2 2
  spline S202 degree 2 poles (31.0423, -21.1) (31.3253, -20.9604) (31.7815, -20.5258) (32.0315, -20.1433) knots 0 0 0 1 2 2 2
  line L215 (32.0315, -20.1433) -> (32.3131, -19.7126)
  line L216 (32.3131, -19.7126) -> (29.0395, -17.5728)
  line L217 (29.0395, -17.5728) -> (28.758, -18.0035)
  spline S203 degree 2 poles (28.758, -18.0035) (28.5125, -18.3791) (28.2614, -19.0265) (28.2725, -19.3633) knots 0 0 0 1 2 2 2
  spline S204 degree 2 poles (28.2725, -19.3633) (28.2786, -19.7903) (28.7465, -20.5191) (29.2427, -20.8434) knots 0 0 0 1 2 2 2
  line L218 (25.8506, -21.0532) -> (26.2514, -20.5514)
  line L219 (26.2514, -20.5514) -> (29.2302, -22.9301)
  line L220 (29.2302, -22.9301) -> (28.8295, -23.4319)
  line L221 (28.8295, -23.4319) -> (25.8506, -21.0532)
  line L222 (29.2966, -23.8629) -> (29.7513, -23.2935)
  line L223 (29.7513, -23.2935) -> (30.2725, -23.7096)
  line L224 (30.2725, -23.7096) -> (29.8178, -24.279)
  line L225 (29.8178, -24.279) -> (29.2966, -23.8629)
  spline S205 degree 2 poles (24.1081, -23.6182) (24.1196, -23.5217) (24.1494, -23.1887) (24.1888, -23.0564) knots 0 0 0 1 2 2 2
  spline S206 degree 2 poles (24.1888, -23.0564) (24.2381, -22.8713) (24.3857, -22.5752) (24.5827, -22.3649) knots 0 0 0 1 2 2 2
  spline S207 degree 2 poles (24.5827, -22.3649) (24.7431, -22.1936) (25.1622, -22.0052) (25.3891, -21.9978) knots 0 0 0 1 2 2 2
  spline S208 degree 2 poles (25.3891, -21.9978) (25.6074, -21.9936) (26.0706, -22.1736) (26.2569, -22.3481) knots 0 0 0 1 2 2 2
  spline S209 degree 2 poles (26.2569, -22.3481) (26.5453, -22.6182) (26.7259, -23.2444) (26.5954, -23.6185) knots 0 0 0 1 2 2 2
  spline S210 degree 2 poles (26.5954, -23.6185) (26.4841, -23.9542) (25.9685, -24.6671) (25.6434, -25.0563) knots 0 0 0 1 2 2 2
  line L226 (25.6434, -25.0563) -> (25.7335, -25.1408)
  spline S211 degree 2 poles (25.7335, -25.1408) (25.8958, -25.2927) (26.1899, -25.3822) (26.3315, -25.3455) knots 0 0 0 1 2 2 2
  spline S212 degree 2 poles (26.3315, -25.3455) (26.473, -25.3088) (26.7511, -25.0842) (26.8805, -24.946) knots 0 0 0 1 2 2 2
  spline S213 degree 2 poles (26.8805, -24.946) (27.0325, -24.7838) (27.3472, -24.2551) (27.4596, -23.9485) knots 0 0 0 1 2 2 2
  line L227 (27.4596, -23.9485) -> (27.4849, -23.9215)
  line L228 (27.4849, -23.9215) -> (27.9626, -24.369)
  spline S214 degree 2 poles (27.9626, -24.369) (27.8776, -24.5319) (27.5146, -25.1001) (27.2923, -25.3374) knots 0 0 0 1 2 2 2
  spline S215 degree 2 poles (27.2923, -25.3374) (27.0221, -25.6258) (26.5633, -25.935) (26.2998, -25.9815) knots 0 0 0 1 2 2 2
  spline S216 degree 2 poles (26.2998, -25.9815) (26.0421, -26.0277) (25.5378, -25.8374) (25.2765, -25.5926) knots 0 0 0 1 2 2 2
  line L229 (25.2765, -25.5926) -> (23.3747, -23.8111)
  line L230 (23.3747, -23.8111) -> (23.8137, -23.3424)
  line L231 (23.8137, -23.3424) -> (24.1081, -23.6182)
  line L232 (24.4987, -23.9841) -> (25.2708, -24.7074)
  spline S217 degree 2 poles (25.2708, -24.7074) (25.4134, -24.525) (25.838, -23.9694) (25.9391, -23.7652) knots 0 0 0 1 2 2 2
  spline S218 degree 2 poles (25.9391, -23.7652) (26.0565, -23.5254) (26.0471, -23.0597) (25.8368, -22.8627) knots 0 0 0 1 2 2 2
  spline S219 degree 2 poles (25.8368, -22.8627) (25.5964, -22.6376) (25.0998, -22.68) (24.8577, -22.9384) knots 0 0 0 1 2 2 2
  spline S220 degree 2 poles (24.8577, -22.9384) (24.6523, -23.1577) (24.5039, -23.6956) (24.4987, -23.9841) knots 0 0 0 1 2 2 2
  line L233 (19.3937, -27.1793) -> (20.7732, -28.9015)
  spline S221 degree 2 poles (20.7732, -28.9015) (20.9379, -29.1071) (21.2505, -29.4316) (21.3791, -29.4868) knots 0 0 0 1 2 2 2
  spline S222 degree 2 poles (21.3791, -29.4868) (21.5155, -29.5517) (21.7938, -29.4975) (21.9641, -29.3611) knots 0 0 0 1 2 2 2
  spline S223 degree 2 poles (21.9641, -29.3611) (22.1183, -29.2376) (22.3199, -28.7649) (22.3622, -28.4357) knots 0 0 0 1 2 2 2
  spline S224 degree 2 poles (22.3622, -28.4357) (22.3229, -28.3933) (22.2161, -28.2731) (22.1492, -28.1896) knots 0 0 0 1 2 2 2
  line L234 (22.1492, -28.1896) -> (20.5793, -26.2296)
  line L235 (20.5793, -26.2296) -> (21.0806, -25.8281)
  line L236 (21.0806, -25.8281) -> (22.46, -27.5503)
  spline S225 degree 2 poles (22.46, -27.5503) (22.6247, -27.756) (22.9374, -28.0805) (23.066, -28.1357) knots 0 0 0 1 2 2 2
  spline S226 degree 2 poles (23.066, -28.1357) (23.2023, -28.2005) (23.4807, -28.1464) (23.651, -28.01) knots 0 0 0 1 2 2 2
  spline S227 degree 2 poles (23.651, -28.01) (23.8116, -27.8813) (24.0061, -27.3932) (24.0471, -27.1019) knots 0 0 0 1 2 2 2
  line L237 (24.0471, -27.1019) -> (22.2662, -24.8785)
  line L238 (22.2662, -24.8785) -> (22.7674, -24.477)
  line L239 (22.7674, -24.477) -> (25.1506, -27.4523)
  line L240 (25.1506, -27.4523) -> (24.6493, -27.8538)
  line L241 (24.6493, -27.8538) -> (24.3868, -27.5261)
  spline S228 degree 2 poles (24.3868, -27.5261) (24.3478, -27.879) (24.1347, -28.4031) (23.9033, -28.5884) knots 0 0 0 1 2 2 2
  spline S229 degree 2 poles (23.9033, -28.5884) (23.6399, -28.7995) (23.0388, -28.8853) (22.714, -28.6972) knots 0 0 0 1 2 2 2
  spline S230 degree 2 poles (22.714, -28.6972) (22.6892, -29.1337) (22.4671, -29.7388) (22.2165, -29.9396) knots 0 0 0 1 2 2 2
  spline S231 degree 2 poles (22.2165, -29.9396) (22.0237, -30.094) (21.6136, -30.2273) (21.3898, -30.185) knots 0 0 0 1 2 2 2
  spline S232 degree 2 poles (21.3898, -30.185) (21.1629, -30.1453) (20.7068, -29.846) (20.4624, -29.5407) knots 0 0 0 1 2 2 2
  line L242 (20.4624, -29.5407) -> (18.8925, -27.5807)
  line L243 (18.8925, -27.5807) -> (19.3937, -27.1793)
  line L244 (18.5793, -31.0455) -> (19.274, -30.6191)
  line L245 (19.274, -30.6191) -> (19.7823, -31.4471)
  line L246 (19.7823, -31.4471) -> (19.0876, -31.8735)
  line L247 (19.0876, -31.8735) -> (18.5793, -31.0455)
  line L248 (17.0933, -28.6247) -> (17.788, -28.1983)
  line L249 (17.788, -28.1983) -> (18.2962, -29.0263)
  line L250 (18.2962, -29.0263) -> (17.6016, -29.4527)
  line L251 (17.6016, -29.4527) -> (17.0933, -28.6247)
  line L252 (11.4641, -31.3331) -> (13.7553, -30.3887)
  line L253 (13.7553, -30.3887) -> (13.953, -30.8682)
  line L254 (13.953, -30.8682) -> (13.1004, -31.2197)
  line L255 (13.1004, -31.2197) -> (14.3979, -34.3672)
  line L256 (14.3979, -34.3672) -> (15.2504, -34.0158)
  line L257 (15.2504, -34.0158) -> (15.4277, -34.4459)
  spline S233 degree 2 poles (15.4277, -34.4459) (14.9444, -34.6451) (14.6006, -35.1074) (14.727, -35.5006) knots 0 0 0 1 2 2 2
  line L258 (14.727, -35.5006) -> (14.2399, -35.7014)
  line L259 (14.2399, -35.7014) -> (12.4953, -31.4691)
  line L260 (12.4953, -31.4691) -> (11.6618, -31.8127)
  line L261 (11.6618, -31.8127) -> (11.4641, -31.3331)
  line L262 (9.5351, -31.9474) -> (10.3133, -31.7048)
  line L263 (10.3133, -31.7048) -> (10.6024, -32.6323)
  line L264 (10.6024, -32.6323) -> (9.8242, -32.8749)
  line L265 (9.8242, -32.8749) -> (9.5351, -31.9474)
  spline S234 degree 2 poles (5.8903, -34.4859) (5.8127, -34.1278) (5.9096, -33.4666) (6.07, -33.196) knots 0 0 0 1 2 2 2
  spline S235 degree 2 poles (6.07, -33.196) (6.2304, -32.9253) (6.7974, -32.5287) (7.1836, -32.4451) knots 0 0 0 1 2 2 2
  spline S236 degree 2 poles (7.1836, -32.4451) (7.5377, -32.3684) (8.2637, -32.3754) (8.5442, -32.4452) knots 0 0 0 1 2 2 2
  line L266 (8.5442, -32.4452) -> (8.6967, -33.1493)
  line L267 (8.6967, -33.1493) -> (8.6484, -33.1598)
  spline S237 degree 2 poles (8.6484, -33.1598) (8.5598, -33.12) (8.2427, -33.037) (8.0558, -33.0101) knots 0 0 0 1 2 2 2
  spline S238 degree 2 poles (8.0558, -33.0101) (7.8438, -32.9844) (7.5014, -32.9786) (7.2962, -33.023) knots 0 0 0 1 2 2 2
  spline S239 degree 2 poles (7.2962, -33.023) (7.095, -33.0666) (6.7482, -33.2934) (6.6454, -33.4799) knots 0 0 0 1 2 2 2
  spline S240 degree 2 poles (6.6454, -33.4799) (6.5529, -33.6558) (6.5096, -34.078) (6.5671, -34.3435) knots 0 0 0 1 2 2 2
  spline S241 degree 2 poles (6.5671, -34.3435) (6.6246, -34.6091) (6.8426, -34.9156) (7.0038, -34.9987) knots 0 0 0 1 2 2 2
  spline S242 degree 2 poles (7.0038, -34.9987) (7.1717, -35.0929) (7.6128, -35.1069) (7.8662, -35.052) knots 0 0 0 1 2 2 2